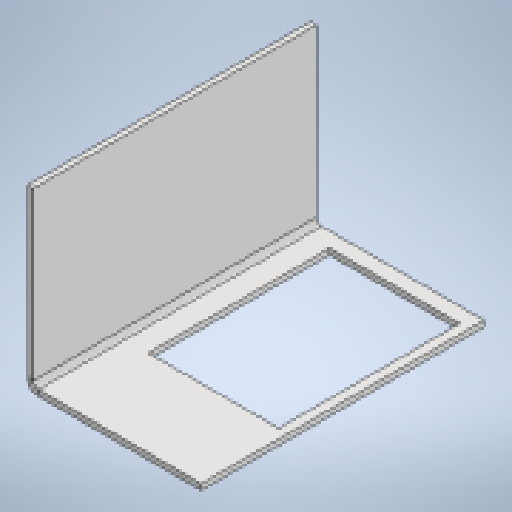
# Autodesk Inventor part: PNS 752 FDS 1200 FLANGE 2
Saved by Autodesk Inventor 2025.3 (Build 293356030, 356C)
## iProperties
Created: 2025-06-24
Part Number: PNS 752 FDS 1200 FLANGE 2
Material: Stainless Steel
Description: DIE16(5)|\ 90°|corrY -___°|X_____|bom___
Document SubType Name: Sheet Metal
Designer: user
Mass: 331.753 g
Surface Area: 434.587 cm^2
Volume: 41.4691 cm^3
Density: 8 g/cm^3
Sheet Metal Rule: AISI304 2mm Die16
Sheet Metal Width: 180,893 mm
Sheet Metal Length: 150,000 mm
Sheet Metal Area: 27133,971 mm^2
Appearance: Default
Flat Pattern Width: 18.0893 cm
Flat Pattern Length: 15 cm
Flat Pattern Area: 271.34 cm^2
Author: user
Autodesk Inventor part; units mm, degrees
ref_plane "YZ Plane" through (0, 0, 0) normal (1, 0, 0) x (0, 1, 0)
ref_plane "XZ Plane" through (0, 0, 0) normal (0, 1, 0) x (-1, 0, 0)
ref_plane "XY Plane" through (0, 0, 0) normal (0, 0, 1) x (1, 0, 0)
sketch "Sketch1" plane through (0, 0, 0) normal (0, 0, 1) x (1, 0, 0)
  line L0 (-46, -75) -> (46, -75)
  line L1 (46, -75) -> (46, 75)
  line L2 (46, 75) -> (-46, 75)
  line L3 (-46, 75) -> (-46, -75)
  line L4 (-46, -75) -> (46, 75) construction
  line L5 (46, -75) -> (-46, 75) construction
  point P0 (0, 0)
  dimension "d154" = 92
  dimension "d155" = 150
  measures "d154" distance of L1.end L2.end
  measures "d155" distance of L0.end L1.end
extrude "Plate5" add sketch "Sketch1" along normal blind 3
sketch "Sketch7" plane through (-43, -75, 0) normal (-1, 0, 0) x (0, -1, 0)
  line L0 (-150, 0) -> (0, 0)
  line L1 (0, 0) -> (0, 94)
  line L2 (0, 94) -> (-150, 94)
  line L3 (-150, 94) -> (-150, 0)
  constraints: 6 end point, 1 horizontal, 1 perpendicular, 1 vertical
edge flange "Flange3" height 94 angle 90 thickness 3 bend radius 2.75 thickness toward (-1, 0, 0) relief round relief width 3 relief depth 1.5 edges at (-46, 0, 3) wall of the first edge with corners at (-43, 75, 0) (-43, -75, 0) (-43, -75, 94) (-43, 75, 94)
bend "Bend3"
corner "Corner3"
sketch "Sketch8" plane through (0, 0, 3) normal (0, 0, 1) x (1, 0, 0)
  line L0 (46, 75) -> (46, -75) projected
  line L1 (-40.25, 75) -> (46, 75) projected
  line L2 (41, 67) -> (-28, 67)
  line L3 (-28, 67) -> (-28, -29)
  line L4 (-28, -29) -> (41, -29)
  line L5 (41, -29) -> (41, 67)
  line L6 (41, 67) -> (-28, -29) construction
  line L7 (-28, 67) -> (41, -29) construction
  line L8 (-40.25, 75) -> (-43, 75) projected
  point P0 (0, 0)
  point P1 (6.5, 19)
  point P2 (2.875, 75)
  point P3 (-41.625, 75)
  dimension "d167" = 69
  dimension "d168" = 96
  dimension "d169" = 8
  dimension "d174" = 13.625
  dimension "d175" = 5
  constraints: 12 end point, 4 midpoint, 2 parallel, 1 horizontal, 1 perpendicular
  measures "d167" distance of L4.end L3.end
  measures "d168" distance of L3.end L2.end
  measures "d169" distance between parallel lines of L1 L2
  measures "d174" distance from line of L3 point (-41.625, 75)
  measures "d175" distance between parallel lines of L0 L5
extrude "Cut1" cut sketch "Sketch8" against normal blind 3
body "Solid3"
